Autodesk Inventor part; units mm, degrees
(part 3 of 4)
  arc A595 (24.0109, 33.4184) -> (24.0599, 33.8093) centre (17.6805, 34.4109) ccw
  arc A596 (24.0599, 33.8093) -> (24.09, 34.2945) centre (16.5061, 34.5221) ccw
  arc A597 (24.09, 34.2945) -> (23.7273, 34.4617) centre (15.3265, 15.7621) ccw
  arc A598 (23.7273, 34.4617) -> (23.3779, 34.1237) centre (28.8257, 28.8427) ccw
  arc A599 (23.3779, 34.1237) -> (23.1125, 33.8326) centre (27.9785, 29.6635) ccw
  arc A600 (23.1125, 33.8326) -> (22.9159, 33.5888) centre (27.1156, 30.4021) ccw
  arc A601 (22.9159, 33.5888) -> (22.5655, 33.7339) centre (15.3265, 15.7621) ccw
  arc A602 (22.5655, 33.7339) -> (22.5988, 34.0453) centre (17.3425, 34.4503) ccw
  arc A603 (22.5988, 34.0453) -> (22.617, 34.4389) centre (16.2101, 34.5381) ccw
  arc A604 (22.617, 34.4389) -> (22.609, 34.9249) centre (15.0306, 34.5568) ccw
  arc A605 (22.609, 34.9249) -> (22.2342, 35.0632) centre (15.3265, 15.7621) ccw
  arc A606 (22.2342, 35.0632) -> (21.9125, 34.6988) centre (27.7578, 29.8615) ccw
  arc A607 (21.9125, 34.6988) -> (21.6707, 34.3877) centre (26.8488, 30.6133) ccw
  arc A608 (21.6707, 34.3877) -> (21.4938, 34.1293) centre (25.9306, 31.2819) ccw
  arc A609 (21.4938, 34.1293) -> (21.1331, 34.2465) centre (15.3265, 15.7621) ccw
  arc A610 (21.1331, 34.2465) -> (21.1419, 34.5595) centre (15.87, 34.5508) ccw
  arc A611 (21.1419, 34.5595) -> (21.1292, 34.9533) centre (14.7342, 34.5495) ccw
  arc A612 (21.1292, 34.9533) -> (21.083, 35.4372) centre (13.5569, 34.4756) ccw
  arc A613 (21.083, 35.4372) -> (20.6986, 35.5457) centre (15.3265, 15.7621) ccw
  arc A614 (20.6986, 35.5457) -> (20.4064, 35.1572) centre (26.6132, 30.7934) ccw
  arc A615 (20.4064, 35.1572) -> (20.1898, 34.8281) centre (25.648, 31.4715) ccw
  arc A616 (20.1898, 34.8281) -> (20.0337, 34.5566) centre (24.6803, 32.0661) ccw
  arc A617 (20.0337, 34.5566) -> (19.6649, 34.6451) centre (15.3265, 15.7621) ccw
  arc A618 (19.6649, 34.6451) -> (19.6491, 34.9579) centre (14.3942, 34.5355) ccw
  arc A619 (19.6491, 34.9579) -> (19.6056, 35.3494) centre (13.262, 34.4452) ccw
  arc A620 (19.6056, 35.3494) -> (19.5216, 35.8282) centre (12.0941, 34.2791) ccw
  arc A621 (19.5216, 35.8282) -> (19.1298, 35.9062) centre (15.3265, 15.7621) ccw
  arc A622 (19.1298, 35.9062) -> (18.869, 35.4959) centre (25.3991, 31.6326) ccw
  arc A623 (18.869, 35.4959) -> (18.6789, 35.1509) centre (24.3837, 32.2329) ccw
  arc A624 (18.6789, 35.1509) -> (18.5446, 34.8679) centre (23.3723, 32.7497) ccw
  arc A625 (18.5446, 34.8679) -> (18.17, 34.9273) centre (15.3265, 15.7621) ccw
  arc A626 (18.17, 34.9273) -> (18.1297, 35.2378) centre (12.9241, 34.4045) ccw
  arc A627 (18.1297, 35.2378) -> (18.0556, 35.6248) centre (11.8025, 34.2256) ccw
  arc A628 (18.0556, 35.6248) -> (17.9343, 36.0955) centre (10.6512, 33.9684) ccw
  arc A629 (17.9343, 36.0955) -> (17.5376, 36.1425) centre (15.3265, 15.7621) ccw
  arc A630 (17.5376, 36.1425) -> (17.3098, 35.713) centre (24.1229, 32.3739) ccw
  arc A631 (17.3098, 35.713) -> (17.1473, 35.3541) centre (23.0635, 32.8927) ccw
  arc A632 (17.1473, 35.3541) -> (17.0357, 35.0615) centre (22.0146, 33.3286) ccw
  arc A633 (17.0357, 35.0615) -> (16.6576, 35.0913) centre (15.3265, 15.7621) ccw
  arc A634 (16.6576, 35.0913) -> (16.593, 35.3977) centre (11.4688, 34.1586) ccw
  arc A635 (16.593, 35.3977) -> (16.4887, 35.7777) centre (10.3647, 33.8922) ccw
  arc A636 (16.4887, 35.7777) -> (16.3309, 36.2374) centre (9.2372, 33.5455) ccw
  arc A637 (16.3309, 36.2374) -> (15.9318, 36.2531) centre (15.3265, 15.7621) ccw
  arc A638 (15.9318, 36.2531) -> (15.7383, 35.8071) centre (22.7924, 33.0129) ccw
  arc A639 (15.7383, 35.8071) -> (15.6046, 35.4366) centre (21.6956, 33.447) ccw
  circle A640 centre (15.3265, 15.7621) radius 18.25
  point P0 (0, 0)
  dimension "d2" = 36.5
  constraints: 1 centre point, 1 coincident
  measures "d2" diameter of A640
extrude "押し出し2" cut sketch "スケッチ2" against normal blind 0.75 contours A640
sketch "スケッチ3" plane through (0, 0, 0) normal (0, 0, -1) x (-1, 0, 0)
  arc A0 (-15.5162, 35.1361) -> (-15.6046, 35.4366) centre (-20.6157, 33.7992) ccw
  arc A1 (-15.6046, 35.4366) -> (-15.7383, 35.8071) centre (-21.6956, 33.447) ccw
  arc A2 (-15.7383, 35.8071) -> (-15.9318, 36.2531) centre (-22.7924, 33.0129) ccw
  arc A3 (-15.9318, 36.2531) -> (-16.3309, 36.2374) centre (-15.3265, 15.7621) ccw
  arc A4 (-16.3309, 36.2374) -> (-16.4887, 35.7777) centre (-9.2372, 33.5455) ccw
  arc A5 (-16.4887, 35.7777) -> (-16.593, 35.3977) centre (-10.3647, 33.8922) ccw
  arc A6 (-16.593, 35.3977) -> (-16.6576, 35.0913) centre (-11.4688, 34.1586) ccw
  arc A7 (-16.6576, 35.0913) -> (-17.0357, 35.0615) centre (-15.3265, 15.7621) ccw
  arc A8 (-17.0357, 35.0615) -> (-17.1473, 35.3541) centre (-22.0146, 33.3286) ccw
  arc A9 (-17.1473, 35.3541) -> (-17.3098, 35.713) centre (-23.0635, 32.8927) ccw
  arc A10 (-17.3098, 35.713) -> (-17.5376, 36.1425) centre (-24.1229, 32.3739) ccw
  arc A11 (-17.5376, 36.1425) -> (-17.9343, 36.0955) centre (-15.3265, 15.7621) ccw
  arc A12 (-17.9343, 36.0955) -> (-18.0556, 35.6248) centre (-10.6512, 33.9684) ccw
  arc A13 (-18.0556, 35.6248) -> (-18.1297, 35.2378) centre (-11.8025, 34.2256) ccw
  arc A14 (-18.1297, 35.2378) -> (-18.17, 34.9273) centre (-12.9241, 34.4045) ccw
  arc A15 (-18.17, 34.9273) -> (-18.5446, 34.8679) centre (-15.3265, 15.7621) ccw
  arc A16 (-18.5446, 34.8679) -> (-18.6789, 35.1509) centre (-23.3723, 32.7497) ccw
  arc A17 (-18.6789, 35.1509) -> (-18.869, 35.4959) centre (-24.3837, 32.2329) ccw
  arc A18 (-18.869, 35.4959) -> (-19.1298, 35.9062) centre (-25.3991, 31.6326) ccw
  arc A19 (-19.1298, 35.9062) -> (-19.5216, 35.8282) centre (-15.3265, 15.7621) ccw
  arc A20 (-19.5216, 35.8282) -> (-19.6056, 35.3494) centre (-12.0941, 34.2791) ccw
  arc A21 (-19.6056, 35.3494) -> (-19.6491, 34.9579) centre (-13.262, 34.4452) ccw
  arc A22 (-19.6491, 34.9579) -> (-19.6649, 34.6451) centre (-14.3942, 34.5355) ccw
  arc A23 (-19.6649, 34.6451) -> (-20.0337, 34.5566) centre (-15.3265, 15.7621) ccw
  arc A24 (-20.0337, 34.5566) -> (-20.1898, 34.8281) centre (-24.6803, 32.0661) ccw
  arc A25 (-20.1898, 34.8281) -> (-20.4064, 35.1572) centre (-25.648, 31.4715) ccw
  arc A26 (-20.4064, 35.1572) -> (-20.6986, 35.5457) centre (-26.6132, 30.7934) ccw
  arc A27 (-20.6986, 35.5457) -> (-21.083, 35.4372) centre (-15.3265, 15.7621) ccw
  arc A28 (-21.083, 35.4372) -> (-21.1292, 34.9533) centre (-13.5569, 34.4756) ccw
  arc A29 (-21.1292, 34.9533) -> (-21.1419, 34.5595) centre (-14.7342, 34.5495) ccw
  arc A30 (-21.1419, 34.5595) -> (-21.1331, 34.2465) centre (-15.87, 34.5508) ccw
  arc A31 (-21.1331, 34.2465) -> (-21.4938, 34.1293) centre (-15.3265, 15.7621) ccw
  arc A32 (-21.4938, 34.1293) -> (-21.6707, 34.3877) centre (-25.9306, 31.2819) ccw
  arc A33 (-21.6707, 34.3877) -> (-21.9125, 34.6988) centre (-26.8488, 30.6133) ccw
  arc A34 (-21.9125, 34.6988) -> (-22.2342, 35.0632) centre (-27.7578, 29.8615) ccw
  arc A35 (-22.2342, 35.0632) -> (-22.609, 34.9249) centre (-15.3265, 15.7621) ccw
  arc A36 (-22.609, 34.9249) -> (-22.617, 34.4389) centre (-15.0306, 34.5568) ccw
  arc A37 (-22.617, 34.4389) -> (-22.5988, 34.0453) centre (-16.2101, 34.5381) ccw
  arc A38 (-22.5988, 34.0453) -> (-22.5655, 33.7339) centre (-17.3425, 34.4503) ccw
  arc A39 (-22.5655, 33.7339) -> (-22.9159, 33.5888) centre (-15.3265, 15.7621) ccw
  arc A40 (-22.9159, 33.5888) -> (-23.1125, 33.8326) centre (-27.1156, 30.4021) ccw
  arc A41 (-23.1125, 33.8326) -> (-23.3779, 34.1237) centre (-27.9785, 29.6635) ccw
  arc A42 (-23.3779, 34.1237) -> (-23.7273, 34.4617) centre (-28.8257, 28.8427) ccw
  arc A43 (-23.7273, 34.4617) -> (-24.09, 34.2945) centre (-15.3265, 15.7621) ccw
  arc A44 (-24.09, 34.2945) -> (-24.0599, 33.8093) centre (-16.5061, 34.5221) ccw
  arc A45 (-24.0599, 33.8093) -> (-24.0109, 33.4184) centre (-17.6805, 34.4109) ccw
  arc A46 (-24.0109, 33.4184) -> (-23.9532, 33.1106) centre (-18.8025, 34.2345) ccw
  arc A47 (-23.9532, 33.1106) -> (-24.2911, 32.9384) centre (-15.3265, 15.7621) ccw
  arc A48 (-24.2911, 32.9384) -> (-24.5063, 33.166) centre (-28.2279, 29.432) ccw
  arc A49 (-24.5063, 33.166) -> (-24.7937, 33.4354) centre (-29.0302, 28.628) ccw
  arc A50 (-24.7937, 33.4354) -> (-25.1685, 33.745) centre (-29.8104, 27.7432) ccw
  arc A51 (-25.1685, 33.745) -> (-25.5171, 33.5498) centre (-15.3265, 15.7621) ccw
  arc A52 (-25.5171, 33.5498) -> (-25.449, 33.0685) centre (-17.9744, 34.3717) ccw
  arc A53 (-25.449, 33.0685) -> (-25.3694, 32.6826) centre (-19.1364, 34.1687) ccw
  arc A54 (-25.3694, 32.6826) -> (-25.2878, 32.3803) centre (-20.2411, 33.9048) ccw
  arc A55 (-25.2878, 32.3803) -> (-25.6112, 32.1821) centre (-15.3265, 15.7621) ccw
  arc A56 (-25.6112, 32.1821) -> (-25.8435, 32.3921) centre (-29.2607, 28.3776) ccw
  arc A57 (-25.8435, 32.3921) -> (-26.1512, 32.6381) centre (-29.9974, 27.5131) ccw
  arc A58 (-26.1512, 32.6381) -> (-26.5491, 32.9173) centre (-30.7058, 26.5699) ccw
  arc A59 (-26.5491, 32.9173) -> (-26.8813, 32.6954) centre (-15.3265, 15.7621) ccw
  arc A60 (-26.8813, 32.6954) -> (-26.7756, 32.2209) centre (-19.4263, 34.1066) ccw
  arc A61 (-26.7756, 32.2209) -> (-26.666, 31.8425) centre (-20.5688, 33.8131) ccw
  arc A62 (-26.666, 31.8425) -> (-26.5609, 31.5475) centre (-21.6494, 33.4633) ccw
  arc A63 (-26.5609, 31.5475) -> (-26.8677, 31.3246) centre (-15.3265, 15.7621) ccw
  arc A64 (-26.8677, 31.3246) -> (-27.1158, 31.5157) centre (-30.2075, 27.2455) ccw
  arc A65 (-27.1158, 31.5157) -> (-27.4419, 31.7368) centre (-30.8741, 26.3258) ccw
  arc A66 (-27.4419, 31.7368) -> (-27.8605, 31.984) centre (-31.5063, 25.33) ccw
  arc A67 (-27.8605, 31.984) -> (-28.1742, 31.7366) centre (-15.3265, 15.7621) ccw
  arc A68 (-28.1742, 31.7366) -> (-28.0317, 31.2719) centre (-20.853, 33.7284) ccw
  arc A69 (-28.0317, 31.2719) -> (-27.8927, 30.9032) centre (-21.9689, 33.3461) ccw
  arc A70 (-27.8927, 30.9032) -> (-27.7648, 30.6174) centre (-23.0188, 32.9126) ccw
  arc A71 (-27.7648, 30.6174) -> (-28.0532, 30.3711) centre (-15.3265, 15.7621) ccw
  arc A72 (-28.0532, 30.3711) -> (-28.3155, 30.5421) centre (-31.0626, 26.0425) ccw
  arc A73 (-28.3155, 30.5421) -> (-28.6579, 30.737) centre (-31.655, 25.0734) ccw
  arc A74 (-28.6579, 30.737) -> (-29.0946, 30.9505) centre (-32.2071, 24.031) ccw
  arc A75 (-29.0946, 30.9505) -> (-29.388, 30.6794) centre (-15.3265, 15.7621) ccw
  arc A76 (-29.388, 30.6794) -> (-29.2094, 30.2273) centre (-22.2456, 33.2394) ccw
  arc A77 (-29.2094, 30.2273) -> (-29.0419, 29.8706) centre (-23.3281, 32.7708) ccw
  arc A78 (-29.0419, 29.8706) -> (-28.892, 29.5957) centre (-24.3407, 32.2563) ccw
  arc A79 (-28.892, 29.5957) -> (-29.1602, 29.3275) centre (-15.3265, 15.7621) ccw
  arc A80 (-29.1602, 29.3275) -> (-29.4351, 29.4775) centre (-31.8207, 24.7762) ccw
  arc A81 (-29.4351, 29.4775) -> (-29.7917, 29.6449) centre (-32.3352, 23.7636) ccw
  arc A82 (-29.7917, 29.6449) -> (-30.2439, 29.8235) centre (-32.8039, 22.6811) ccw
  arc A83 (-30.2439, 29.8235) -> (-30.515, 29.5302) centre (-15.3265, 15.7621) ccw
  arc A84 (-30.515, 29.5302) -> (-30.3015, 29.0934) centre (-23.5955, 32.6427) ccw
  arc A85 (-30.3015, 29.0934) -> (-30.1066, 28.751) centre (-24.6379, 32.0905) ccw
  arc A86 (-30.1066, 28.751) -> (-29.9356, 28.4887) centre (-25.607, 31.4982) ccw
  arc A87 (-29.9356, 28.4887) -> (-30.1819, 28.2003) centre (-15.3265, 15.7621) ccw
  arc A88 (-30.1819, 28.2003) -> (-30.4677, 28.3282) centre (-32.4771, 23.4543) ccw
  arc A89 (-30.4677, 28.3282) -> (-30.8364, 28.4672) centre (-32.9106, 22.4045) ccw
  arc A90 (-30.8364, 28.4672) -> (-31.3011, 28.6097) centre (-33.2929, 21.2885) ccw
  arc A91 (-31.3011, 28.6097) -> (-31.5484, 28.296) centre (-15.3265, 15.7621) ccw
  arc A92 (-31.5484, 28.296) -> (-31.3013, 27.8774) centre (-24.8944, 31.9418) ccw
  arc A93 (-31.3013, 27.8774) -> (-31.0801, 27.5514) centre (-25.8903, 31.3096) ccw
  arc A94 (-31.0801, 27.5514) -> (-30.889, 27.3033) centre (-26.81, 30.6431) ccw
  arc A95 (-30.889, 27.3033) -> (-31.112, 26.9964) centre (-15.3265, 15.7621) ccw
  arc A96 (-31.112, 26.9964) -> (-31.407, 27.1015) centre (-33.0278, 22.085) ccw
  arc A97 (-31.407, 27.1015) -> (-31.7854, 27.2111) centre (-33.3775, 21.0044) ccw
  arc A98 (-31.7854, 27.2111) -> (-32.2599, 27.3168) centre (-33.6711, 19.8618) ccw
  arc A99 (-32.2599, 27.3168) -> (-32.4818, 26.9846) centre (-15.3265, 15.7621) ccw
  arc A100 (-32.4818, 26.9846) -> (-32.2026, 26.5867) centre (-26.1344, 31.1413) ccw
  arc A101 (-32.2026, 26.5867) -> (-31.9566, 26.279) centre (-27.0776, 30.4329) ccw
  arc A102 (-31.9566, 26.279) -> (-31.7466, 26.0467) centre (-27.9421, 29.6962) ccw
  arc A103 (-31.7466, 26.0467) -> (-31.9447, 25.7233) centre (-15.3265, 15.7621) ccw
  arc A104 (-31.9447, 25.7233) -> (-32.2471, 25.8049) centre (-33.4693, 20.6766) ccw
  arc A105 (-32.2471, 25.8049) -> (-32.633, 25.8845) centre (-33.7332, 19.5719) ccw
  arc A106 (-32.633, 25.8845) -> (-33.1143, 25.9526) centre (-33.9362, 18.4099) ccw
  arc A107 (-33.1143, 25.9526) -> (-33.3095, 25.6041) centre (-15.3265, 15.7621) ccw
  arc A108 (-33.3095, 25.6041) -> (-32.9999, 25.2293) centre (-27.3077, 30.2459) ccw
  arc A109 (-32.9999, 25.2293) -> (-32.7304, 24.9418) centre (-28.1924, 29.4657) ccw
  arc A110 (-32.7304, 24.9418) -> (-32.5029, 24.7267) centre (-28.9965, 28.6635) ccw
  arc A111 (-32.5029, 24.7267) -> (-32.6751, 24.3888) centre (-15.3265, 15.7621) ccw
  arc A112 (-32.6751, 24.3888) -> (-32.9829, 24.4464) centre (-33.799, 19.238) ccw
  arc A113 (-32.9829, 24.4464) -> (-33.3738, 24.4954) centre (-33.9754, 18.116) ccw
  arc A114 (-33.3738, 24.4954) -> (-33.859, 24.5256) centre (-34.0866, 16.9417) ccw
  arc A115 (-33.859, 24.5256) -> (-34.0262, 24.1628) centre (-15.3265, 15.7621) ccw
  arc A116 (-34.0262, 24.1628) -> (-33.6882, 23.8134) centre (-28.4072, 29.2612) ccw
  arc A117 (-33.6882, 23.8134) -> (-33.397, 23.548) centre (-29.228, 28.414) ccw
  arc A118 (-33.397, 23.548) -> (-33.1533, 23.3514) centre (-29.9666, 27.5512) ccw
  arc A119 (-33.1533, 23.3514) -> (-33.2984, 23.001) centre (-15.3265, 15.7621) ccw
  arc A120 (-33.2984, 23.001) -> (-33.6098, 23.0343) centre (-34.0147, 17.778) ccw
  arc A121 (-33.6098, 23.0343) -> (-34.0034, 23.0525) centre (-34.1026, 16.6456) ccw
  arc A122 (-34.0034, 23.0525) -> (-34.4894, 23.0445) centre (-34.1213, 15.4661) ccw
  arc A123 (-34.4894, 23.0445) -> (-34.6277, 22.6697) centre (-15.3265, 15.7621) ccw
  arc A124 (-34.6277, 22.6697) -> (-34.2633, 22.348) centre (-29.426, 28.1933) ccw
  arc A125 (-34.2633, 22.348) -> (-33.9522, 22.1062) centre (-30.1778, 27.2843) ccw
  arc A126 (-33.9522, 22.1062) -> (-33.6938, 21.9293) centre (-30.8464, 26.3662) ccw
  arc A127 (-33.6938, 21.9293) -> (-33.811, 21.5686) centre (-15.3265, 15.7621) ccw
  arc A128 (-33.811, 21.5686) -> (-34.124, 21.5774) centre (-34.1153, 16.3055) ccw
  arc A129 (-34.124, 21.5774) -> (-34.5178, 21.5647) centre (-34.114, 15.1697) ccw
  arc A130 (-34.5178, 21.5647) -> (-35.0017, 21.5186) centre (-34.0401, 13.9924) ccw
  arc A131 (-35.0017, 21.5186) -> (-35.1102, 21.1341) centre (-15.3265, 15.7621) ccw
  arc A132 (-35.1102, 21.1341) -> (-34.7216, 20.8419) centre (-30.3579, 27.0488) ccw
  arc A133 (-34.7216, 20.8419) -> (-34.3925, 20.6253) centre (-31.036, 26.0836) ccw
  arc A134 (-34.3925, 20.6253) -> (-34.121, 20.4692) centre (-31.6305, 25.1158) ccw
  arc A135 (-34.121, 20.4692) -> (-34.2096, 20.1005) centre (-15.3265, 15.7621) ccw
  arc A136 (-34.2096, 20.1005) -> (-34.5223, 20.0847) centre (-34.1, 14.8297) ccw
  arc A137 (-34.5223, 20.0847) -> (-34.9139, 20.0411) centre (-34.0096, 13.6975) ccw
  arc A138 (-34.9139, 20.0411) -> (-35.3927, 19.9571) centre (-33.8436, 12.5296) ccw
  arc A139 (-35.3927, 19.9571) -> (-35.4707, 19.5653) centre (-15.3265, 15.7621) ccw
  arc A140 (-35.4707, 19.5653) -> (-35.0604, 19.3045) centre (-31.1971, 25.8346) ccw
  arc A141 (-35.0604, 19.3045) -> (-34.7153, 19.1144) centre (-31.7974, 24.8192) ccw
  arc A142 (-34.7153, 19.1144) -> (-34.4324, 18.9801) centre (-32.3142, 23.8078) ccw
  arc A143 (-34.4324, 18.9801) -> (-34.4918, 18.6055) centre (-15.3265, 15.7621) ccw
  arc A144 (-34.4918, 18.6055) -> (-34.8023, 18.5653) centre (-33.969, 13.3596) ccw
  arc A145 (-34.8023, 18.5653) -> (-35.1893, 18.4911) centre (-33.7901, 12.238) ccw
  arc A146 (-35.1893, 18.4911) -> (-35.66, 18.3698) centre (-33.5329, 11.0868) ccw
  arc A147 (-35.66, 18.3698) -> (-35.707, 17.9731) centre (-15.3265, 15.7621) ccw
  arc A148 (-35.707, 17.9731) -> (-35.2775, 17.7453) centre (-31.9384, 24.5584) ccw
  arc A149 (-35.2775, 17.7453) -> (-34.9186, 17.5829) centre (-32.4572, 23.499) ccw
  arc A150 (-34.9186, 17.5829) -> (-34.626, 17.4712) centre (-32.8931, 22.4501) ccw
  arc A151 (-34.626, 17.4712) -> (-34.6558, 17.0931) centre (-15.3265, 15.7621) ccw
  arc A152 (-34.6558, 17.0931) -> (-34.9622, 17.0286) centre (-33.723, 11.9043) ccw
  arc A153 (-34.9622, 17.0286) -> (-35.3421, 16.9243) centre (-33.4566, 10.8002) ccw
  arc A154 (-35.3421, 16.9243) -> (-35.8019, 16.7664) centre (-33.11, 9.6727) ccw
  arc A155 (-35.8019, 16.7664) -> (-35.8176, 16.3673) centre (-15.3265, 15.7621) ccw
  arc A156 (-35.8176, 16.3673) -> (-35.3716, 16.1739) centre (-32.5774, 23.2279) ccw
  arc A157 (-35.3716, 16.1739) -> (-35.0011, 16.0401) centre (-33.0115, 22.1311) ccw
  arc A158 (-35.0011, 16.0401) -> (-34.7006, 15.9517) centre (-33.3636, 21.0513) ccw
  arc A159 (-34.7006, 15.9517) -> (-34.7006, 15.5724) centre (-15.3265, 15.7621) ccw
  arc A160 (-34.7006, 15.5724) -> (-35.0011, 15.4841) centre (-33.3636, 10.4729) ccw
  arc A161 (-35.0011, 15.4841) -> (-35.3716, 15.3503) centre (-33.0115, 9.3931) ccw
  arc A162 (-35.3716, 15.3503) -> (-35.8176, 15.1569) centre (-32.5774, 8.2962) ccw
  arc A163 (-35.8176, 15.1569) -> (-35.8019, 14.7577) centre (-15.3265, 15.7621) ccw
  arc A164 (-35.8019, 14.7577) -> (-35.3421, 14.5999) centre (-33.11, 21.8514) ccw
  arc A165 (-35.3421, 14.5999) -> (-34.9622, 14.4956) centre (-33.4566, 20.7239) ccw
  arc A166 (-34.9622, 14.4956) -> (-34.6558, 14.431) centre (-33.723, 19.6198) ccw
  arc A167 (-34.6558, 14.431) -> (-34.626, 14.053) centre (-15.3265, 15.7621) ccw
  arc A168 (-34.626, 14.053) -> (-34.9186, 13.9413) centre (-32.8931, 9.074) ccw
  arc A169 (-34.9186, 13.9413) -> (-35.2775, 13.7788) centre (-32.4572, 8.0251) ccw
  arc A170 (-35.2775, 13.7788) -> (-35.707, 13.551) centre (-31.9384, 6.9657) ccw
  arc A171 (-35.707, 13.551) -> (-35.66, 13.1543) centre (-15.3265, 15.7621) ccw
  arc A172 (-35.66, 13.1543) -> (-35.1893, 13.033) centre (-33.5329, 20.4374) ccw
  arc A173 (-35.1893, 13.033) -> (-34.8023, 12.9589) centre (-33.7901, 19.2861) ccw
  arc A174 (-34.8023, 12.9589) -> (-34.4918, 12.9186) centre (-33.969, 18.1645) ccw
  arc A175 (-34.4918, 12.9186) -> (-34.4324, 12.544) centre (-15.3265, 15.7621) ccw
  arc A176 (-34.4324, 12.544) -> (-34.7153, 12.4097) centre (-32.3142, 7.7164) ccw
  arc A177 (-34.7153, 12.4097) -> (-35.0604, 12.2196) centre (-31.7974, 6.7049) ccw
  arc A178 (-35.0604, 12.2196) -> (-35.4707, 11.9588) centre (-31.1971, 5.6895) ccw
  arc A179 (-35.4707, 11.9588) -> (-35.3927, 11.567) centre (-15.3265, 15.7621) ccw
  arc A180 (-35.3927, 11.567) -> (-34.9139, 11.4831) centre (-33.8436, 18.9945) ccw
  arc A181 (-34.9139, 11.4831) -> (-34.5223, 11.4395) centre (-34.0096, 17.8266) ccw
  arc A182 (-34.5223, 11.4395) -> (-34.2096, 11.4237) centre (-34.1, 16.6945) ccw
  arc A183 (-34.2096, 11.4237) -> (-34.121, 11.0549) centre (-15.3265, 15.7621) ccw
  arc A184 (-34.121, 11.0549) -> (-34.3925, 10.8988) centre (-31.6305, 6.4083) ccw
  arc A185 (-34.3925, 10.8988) -> (-34.7216, 10.6822) centre (-31.036, 5.4406) ccw
  arc A186 (-34.7216, 10.6822) -> (-35.1102, 10.39) centre (-30.3579, 4.4754) ccw
  arc A187 (-35.1102, 10.39) -> (-35.0017, 10.0056) centre (-15.3265, 15.7621) ccw
  arc A188 (-35.0017, 10.0056) -> (-34.5178, 9.9594) centre (-34.0401, 17.5317) ccw
  arc A189 (-34.5178, 9.9594) -> (-34.124, 9.9467) centre (-34.114, 16.3544) ccw
  arc A190 (-34.124, 9.9467) -> (-33.811, 9.9555) centre (-34.1153, 15.2186) ccw
  arc A191 (-33.811, 9.9555) -> (-33.6938, 9.5948) centre (-15.3265, 15.7621) ccw
  arc A192 (-33.6938, 9.5948) -> (-33.9522, 9.4179) centre (-30.8464, 5.158) ccw
  arc A193 (-33.9522, 9.4179) -> (-34.2633, 9.1762) centre (-30.1778, 4.2398) ccw
  arc A194 (-34.2633, 9.1762) -> (-34.6277, 8.8544) centre (-29.426, 3.3308) ccw
  arc A195 (-34.6277, 8.8544) -> (-34.4894, 8.4796) centre (-15.3265, 15.7621) ccw
  arc A196 (-34.4894, 8.4796) -> (-34.0034, 8.4716) centre (-34.1213, 16.058) ccw
  arc A197 (-34.0034, 8.4716) -> (-33.6098, 8.4898) centre (-34.1026, 14.8785) ccw
  arc A198 (-33.6098, 8.4898) -> (-33.2984, 8.5231) centre (-34.0147, 13.7462) ccw
  arc A199 (-33.2984, 8.5231) -> (-33.1533, 8.1727) centre (-15.3265, 15.7621) ccw
  arc A200 (-33.1533, 8.1727) -> (-33.397, 7.9761) centre (-29.9666, 3.973) ccw
  arc A201 (-33.397, 7.9761) -> (-33.6882, 7.7107) centre (-29.228, 3.1101) ccw
  arc A202 (-33.6882, 7.7107) -> (-34.0262, 7.3613) centre (-28.4072, 2.2629) ccw
  arc A203 (-34.0262, 7.3613) -> (-33.859, 6.9986) centre (-15.3265, 15.7621) ccw
  arc A204 (-33.859, 6.9986) -> (-33.3738, 7.0287) centre (-34.0866, 14.5825) ccw
  arc A205 (-33.3738, 7.0287) -> (-32.9829, 7.0777) centre (-33.9754, 13.4081) ccw
  arc A206 (-32.9829, 7.0777) -> (-32.6751, 7.1354) centre (-33.799, 12.2861) ccw
  arc A207 (-32.6751, 7.1354) -> (-32.5029, 6.7975) centre (-15.3265, 15.7621) ccw
  arc A208 (-32.5029, 6.7975) -> (-32.7304, 6.5823) centre (-28.9965, 2.8607) ccw
  arc A209 (-32.7304, 6.5823) -> (-32.9999, 6.2949) centre (-28.1924, 2.0585) ccw
  arc A210 (-32.9999, 6.2949) -> (-33.3095, 5.9201) centre (-27.3077, 1.2782) ccw
  arc A211 (-33.3095, 5.9201) -> (-33.1143, 5.5715) centre (-15.3265, 15.7621) ccw
  arc A212 (-33.1143, 5.5715) -> (-32.633, 5.6397) centre (-33.9362, 13.1142) ccw
  arc A213 (-32.633, 5.6397) -> (-32.2471, 5.7192) centre (-33.7332, 11.9522) ccw
  arc A214 (-32.2471, 5.7192) -> (-31.9447, 5.8008) centre (-33.4693, 10.8475) ccw
  arc A215 (-31.9447, 5.8008) -> (-31.7466, 5.4775) centre (-15.3265, 15.7621) ccw
  arc A216 (-31.7466, 5.4775) -> (-31.9566, 5.2451) centre (-27.9421, 1.8279) ccw
  arc A217 (-31.9566, 5.2451) -> (-32.2026, 4.9374) centre (-27.0776, 1.0913) ccw
  arc A218 (-32.2026, 4.9374) -> (-32.4818, 4.5395) centre (-26.1344, 0.3829) ccw
  arc A219 (-32.4818, 4.5395) -> (-32.2599, 4.2073) centre (-15.3265, 15.7621) ccw
  arc A220 (-32.2599, 4.2073) -> (-31.7854, 4.313) centre (-33.6711, 11.6623) ccw
  arc A221 (-31.7854, 4.313) -> (-31.407, 4.4226) centre (-33.3775, 10.5198) ccw
  arc A222 (-31.407, 4.4226) -> (-31.112, 4.5277) centre (-33.0278, 9.4392) ccw
  arc A223 (-31.112, 4.5277) -> (-30.889, 4.2209) centre (-15.3265, 15.7621) ccw
  arc A224 (-30.889, 4.2209) -> (-31.0801, 3.9728) centre (-26.81, 0.8811) ccw
  arc A225 (-31.0801, 3.9728) -> (-31.3013, 3.6467) centre (-25.8903, 0.2145) ccw
  arc A226 (-31.3013, 3.6467) -> (-31.5484, 3.2281) centre (-24.8944, -0.4177) ccw
  arc A227 (-31.5484, 3.2281) -> (-31.3011, 2.9144) centre (-15.3265, 15.7621) ccw
  arc A228 (-31.3011, 2.9144) -> (-30.8364, 3.057) centre (-33.2929, 10.2356) ccw
  arc A229 (-30.8364, 3.057) -> (-30.4677, 3.1959) centre (-32.9106, 9.1197) ccw
  arc A230 (-30.4677, 3.1959) -> (-30.1819, 3.3238) centre (-32.4771, 8.0698) ccw
  arc A231 (-30.1819, 3.3238) -> (-29.9356, 3.0354) centre (-15.3265, 15.7621) ccw
  arc A232 (-29.9356, 3.0354) -> (-30.1066, 2.7731) centre (-25.607, 0.026) ccw
  arc A233 (-30.1066, 2.7731) -> (-30.3015, 2.4307) centre (-24.6379, -0.5664) ccw
  arc A234 (-30.3015, 2.4307) -> (-30.515, 1.994) centre (-23.5955, -1.1185) ccw
  arc A235 (-30.515, 1.994) -> (-30.2439, 1.7006) centre (-15.3265, 15.7621) ccw
  arc A236 (-30.2439, 1.7006) -> (-29.7917, 1.8792) centre (-32.8039, 8.843) ccw
  arc A237 (-29.7917, 1.8792) -> (-29.4351, 2.0467) centre (-32.3352, 7.7605) ccw
  arc A238 (-29.4351, 2.0467) -> (-29.1602, 2.1966) centre (-31.8207, 6.7479) ccw
  arc A239 (-29.1602, 2.1966) -> (-28.892, 1.9284) centre (-15.3265, 15.7621) ccw
  arc A240 (-28.892, 1.9284) -> (-29.0419, 1.6535) centre (-24.3407, -0.7321) ccw
  arc A241 (-29.0419, 1.6535) -> (-29.2094, 1.2969) centre (-23.3281, -1.2466) ccw
  arc A242 (-29.2094, 1.2969) -> (-29.388, 0.8447) centre (-22.2456, -1.7153) ccw
  arc A243 (-29.388, 0.8447) -> (-29.0946, 0.5736) centre (-15.3265, 15.7621) ccw
  arc A244 (-29.0946, 0.5736) -> (-28.6579, 0.7871) centre (-32.2071, 7.4931) ccw
  arc A245 (-28.6579, 0.7871) -> (-28.3155, 0.982) centre (-31.655, 6.4507) ccw
  arc A246 (-28.3155, 0.982) -> (-28.0532, 1.1531) centre (-31.0626, 5.4816) ccw
  arc A247 (-28.0532, 1.1531) -> (-27.7648, 0.9068) centre (-15.3265, 15.7621) ccw
  arc A248 (-27.7648, 0.9068) -> (-27.8927, 0.6209) centre (-23.0188, -1.3885) ccw
  arc A249 (-27.8927, 0.6209) -> (-28.0317, 0.2522) centre (-21.9689, -1.822) ccw
  arc A250 (-28.0317, 0.2522) -> (-28.1742, -0.2125) centre (-20.853, -2.2042) ccw
  arc A251 (-28.1742, -0.2125) -> (-27.8605, -0.4598) centre (-15.3265, 15.7621) ccw
  arc A252 (-27.8605, -0.4598) -> (-27.4419, -0.2127) centre (-31.5063, 6.1942) ccw
  arc A253 (-27.4419, -0.2127) -> (-27.1158, 0.0085) centre (-30.8741, 5.1983) ccw
  arc A254 (-27.1158, 0.0085) -> (-26.8677, 0.1996) centre (-30.2075, 4.2787) ccw
  arc A255 (-26.8677, 0.1996) -> (-26.5609, -0.0233) centre (-15.3265, 15.7621) ccw
  arc A256 (-26.5609, -0.0233) -> (-26.666, -0.3184) centre (-21.6494, -1.9392) ccw
  arc A257 (-26.666, -0.3184) -> (-26.7756, -0.6968) centre (-20.5688, -2.2889) ccw
  arc A258 (-26.7756, -0.6968) -> (-26.8813, -1.1713) centre (-19.4263, -2.5825) ccw
  arc A259 (-26.8813, -1.1713) -> (-26.5491, -1.3932) centre (-15.3265, 15.7621) ccw
  arc A260 (-26.5491, -1.3932) -> (-26.1512, -1.114) centre (-30.7058, 4.9542) ccw
  arc A261 (-26.1512, -1.114) -> (-25.8435, -0.868) centre (-29.9974, 4.011) ccw
  arc A262 (-25.8435, -0.868) -> (-25.6112, -0.658) centre (-29.2607, 3.1465) ccw
  arc A263 (-25.6112, -0.658) -> (-25.2878, -0.8561) centre (-15.3265, 15.7621) ccw
  arc A264 (-25.2878, -0.8561) -> (-25.3694, -1.1585) centre (-20.2411, -2.3807) ccw
  arc A265 (-25.3694, -1.1585) -> (-25.449, -1.5443) centre (-19.1364, -2.6446) ccw
  arc A266 (-25.449, -1.5443) -> (-25.5171, -2.0257) centre (-17.9744, -2.8476) ccw
  arc A267 (-25.5171, -2.0257) -> (-25.1685, -2.2208) centre (-15.3265, 15.7621) ccw
  arc A268 (-25.1685, -2.2208) -> (-24.7937, -1.9113) centre (-29.8104, 3.7809) ccw
  arc A269 (-24.7937, -1.9113) -> (-24.5063, -1.6418) centre (-29.0302, 2.8962) ccw
  arc A270 (-24.5063, -1.6418) -> (-24.2911, -1.4143) centre (-28.2279, 2.0921) ccw
  arc A271 (-24.2911, -1.4143) -> (-23.9532, -1.5864) centre (-15.3265, 15.7621) ccw
  arc A272 (-23.9532, -1.5864) -> (-24.0109, -1.8943) centre (-18.8025, -2.7104) ccw
  arc A273 (-24.0109, -1.8943) -> (-24.0599, -2.2852) centre (-17.6805, -2.8868) ccw
  arc A274 (-24.0599, -2.2852) -> (-24.09, -2.7704) centre (-16.5061, -2.998) ccw
  arc A275 (-24.09, -2.7704) -> (-23.7273, -2.9376) centre (-15.3265, 15.7621) ccw
  arc A276 (-23.7273, -2.9376) -> (-23.3779, -2.5996) centre (-28.8257, 2.6814) ccw
  arc A277 (-23.3779, -2.5996) -> (-23.1125, -2.3084) centre (-27.9785, 1.8607) ccw
  arc A278 (-23.1125, -2.3084) -> (-22.9159, -2.0647) centre (-27.1156, 1.122) ccw
  arc A279 (-22.9159, -2.0647) -> (-22.5655, -2.2098) centre (-15.3265, 15.7621) ccw
  arc A280 (-22.5655, -2.2098) -> (-22.5988, -2.5212) centre (-17.3425, -2.9261) ccw
  arc A281 (-22.5988, -2.5212) -> (-22.617, -2.9148) centre (-16.2101, -3.014) ccw
  arc A282 (-22.617, -2.9148) -> (-22.609, -3.4008) centre (-15.0306, -3.0327) ccw
  arc A283 (-22.609, -3.4008) -> (-22.2342, -3.5391) centre (-15.3265, 15.7621) ccw
  arc A284 (-22.2342, -3.5391) -> (-21.9125, -3.1747) centre (-27.7578, 1.6626) ccw
  arc A285 (-21.9125, -3.1747) -> (-21.6707, -2.8636) centre (-26.8488, 0.9109) ccw
  arc A286 (-21.6707, -2.8636) -> (-21.4938, -2.6052) centre (-25.9306, 0.2422) ccw
  arc A287 (-21.4938, -2.6052) -> (-21.1331, -2.7224) centre (-15.3265, 15.7621) ccw
  arc A288 (-21.1331, -2.7224) -> (-21.1419, -3.0354) centre (-15.87, -3.0267) ccw
  arc A289 (-21.1419, -3.0354) -> (-21.1292, -3.4292) centre (-14.7342, -3.0254) ccw
  arc A290 (-21.1292, -3.4292) -> (-21.083, -3.9131) centre (-13.5569, -2.9515) ccw
  arc A291 (-21.083, -3.9131) -> (-20.6986, -4.0215) centre (-15.3265, 15.7621) ccw
  arc A292 (-20.6986, -4.0215) -> (-20.4064, -3.633) centre (-26.6132, 0.7308) ccw
  arc A293 (-20.4064, -3.633) -> (-20.1898, -3.3039) centre (-25.648, 0.0526) ccw
  arc A294 (-20.1898, -3.3039) -> (-20.0337, -3.0324) centre (-24.6803, -0.5419) ccw
  arc A295 (-20.0337, -3.0324) -> (-19.6649, -3.121) centre (-15.3265, 15.7621) ccw
  arc A296 (-19.6649, -3.121) -> (-19.6491, -3.4337) centre (-14.3942, -3.0114) ccw
  arc A297 (-19.6491, -3.4337) -> (-19.6056, -3.8253) centre (-13.262, -2.921) ccw
  arc A298 (-19.6056, -3.8253) -> (-19.5216, -4.3041) centre (-12.0941, -2.755) ccw
  arc A299 (-19.5216, -4.3041) -> (-19.1298, -4.382) centre (-15.3265, 15.7621) ccw
  arc A300 (-19.1298, -4.382) -> (-18.869, -3.9718) centre (-25.3991, -0.1085) ccw
  arc A301 (-18.869, -3.9718) -> (-18.6789, -3.6267) centre (-24.3837, -0.7088) ccw
  arc A302 (-18.6789, -3.6267) -> (-18.5446, -3.3438) centre (-23.3723, -1.2256) ccw
  arc A303 (-18.5446, -3.3438) -> (-18.17, -3.4031) centre (-15.3265, 15.7621) ccw
  arc A304 (-18.17, -3.4031) -> (-18.1297, -3.7137) centre (-12.9241, -2.8804) ccw
  arc A305 (-18.1297, -3.7137) -> (-18.0556, -4.1006) centre (-11.8025, -2.7014) ccw
  arc A306 (-18.0556, -4.1006) -> (-17.9343, -4.5714) centre (-10.6512, -2.4443) ccw
  arc A307 (-17.9343, -4.5714) -> (-17.5376, -4.6183) centre (-15.3265, 15.7621) ccw
  arc A308 (-17.5376, -4.6183) -> (-17.3098, -4.1889) centre (-24.1229, -0.8498) ccw
  arc A309 (-17.3098, -4.1889) -> (-17.1473, -3.83) centre (-23.0635, -1.3686) ccw
  arc A310 (-17.1473, -3.83) -> (-17.0357, -3.5374) centre (-22.0146, -1.8045) ccw
  arc A311 (-17.0357, -3.5374) -> (-16.6576, -3.5672) centre (-15.3265, 15.7621) ccw
  arc A312 (-16.6576, -3.5672) -> (-16.593, -3.8736) centre (-11.4688, -2.6344) ccw
  arc A313 (-16.593, -3.8736) -> (-16.4887, -4.2535) centre (-10.3647, -2.368) ccw
  arc A314 (-16.4887, -4.2535) -> (-16.3309, -4.7133) centre (-9.2372, -2.0213) ccw
  arc A315 (-16.3309, -4.7133) -> (-15.9318, -4.729) centre (-15.3265, 15.7621) ccw
  arc A316 (-15.9318, -4.729) -> (-15.7383, -4.283) centre (-22.7924, -1.4888) ccw
  arc A317 (-15.7383, -4.283) -> (-15.6046, -3.9124) centre (-21.6956, -1.9228) ccw
  arc A318 (-15.6046, -3.9124) -> (-15.5162, -3.612) centre (-20.6157, -2.275) ccw
  arc A319 (-15.5162, -3.612) -> (-15.1369, -3.612) centre (-15.3265, 15.7621) ccw
  arc A320 (-15.1369, -3.612) -> (-15.0485, -3.9124) centre (-10.0373, -2.275) ccw
  arc A321 (-15.0485, -3.9124) -> (-14.9147, -4.283) centre (-8.9575, -1.9228) ccw
  arc A322 (-14.9147, -4.283) -> (-14.7213, -4.729) centre (-7.8607, -1.4888) ccw
  arc A323 (-14.7213, -4.729) -> (-14.3222, -4.7133) centre (-15.3265, 15.7621) ccw
  arc A324 (-14.3222, -4.7133) -> (-14.1644, -4.2535) centre (-21.4159, -2.0213) ccw
  arc A325 (-14.1644, -4.2535) -> (-14.0601, -3.8736) centre (-20.2884, -2.368) ccw
  arc A326 (-14.0601, -3.8736) -> (-13.9955, -3.5672) centre (-19.1843, -2.6344) ccw
  arc A327 (-13.9955, -3.5672) -> (-13.6174, -3.5374) centre (-15.3265, 15.7621) ccw
  arc A328 (-13.6174, -3.5374) -> (-13.5057, -3.83) centre (-8.6385, -1.8045) ccw
  arc A329 (-13.5057, -3.83) -> (-13.3433, -4.1889) centre (-7.5896, -1.3686) ccw
  arc A330 (-13.3433, -4.1889) -> (-13.1155, -4.6183) centre (-6.5302, -0.8498) ccw
  arc A331 (-13.1155, -4.6183) -> (-12.7188, -4.5714) centre (-15.3265, 15.7621) ccw
  arc A332 (-12.7188, -4.5714) -> (-12.5975, -4.1006) centre (-20.0019, -2.4443) ccw
  arc A333 (-12.5975, -4.1006) -> (-12.5234, -3.7137) centre (-18.8506, -2.7014) ccw
  arc A334 (-12.5234, -3.7137) -> (-12.4831, -3.4031) centre (-17.729, -2.8804) ccw
  arc A335 (-12.4831, -3.4031) -> (-12.1085, -3.3438) centre (-15.3265, 15.7621) ccw
  arc A336 (-12.1085, -3.3438) -> (-11.9742, -3.6267) centre (-7.2808, -1.2256) ccw
  arc A337 (-11.9742, -3.6267) -> (-11.7841, -3.9718) centre (-6.2694, -0.7088) ccw
  arc A338 (-11.7841, -3.9718) -> (-11.5233, -4.382) centre (-5.254, -0.1085) ccw
  arc A339 (-11.5233, -4.382) -> (-11.1315, -4.3041) centre (-15.3265, 15.7621) ccw
  arc A340 (-11.1315, -4.3041) -> (-11.0475, -3.8253) centre (-18.559, -2.755) ccw
  arc A341 (-11.0475, -3.8253) -> (-11.0039, -3.4337) centre (-17.3911, -2.921) ccw
  arc A342 (-11.0039, -3.4337) -> (-10.9881, -3.121) centre (-16.2589, -3.0114) ccw
  arc A343 (-10.9881, -3.121) -> (-10.6194, -3.0324) centre (-15.3265, 15.7621) ccw
  arc A344 (-10.6194, -3.0324) -> (-10.4633, -3.3039) centre (-5.9728, -0.5419) ccw
  arc A345 (-10.4633, -3.3039) -> (-10.2467, -3.633) centre (-5.005, 0.0526) ccw
  arc A346 (-10.2467, -3.633) -> (-9.9545, -4.0215) centre (-4.0399, 0.7308) ccw
  arc A347 (-9.9545, -4.0215) -> (-9.57, -3.9131) centre (-15.3265, 15.7621) ccw
  arc A348 (-9.57, -3.9131) -> (-9.5239, -3.4292) centre (-17.0962, -2.9515) ccw
  arc A349 (-9.5239, -3.4292) -> (-9.5112, -3.0354) centre (-15.9189, -3.0254) ccw
  arc A350 (-9.5112, -3.0354) -> (-9.52, -2.7224) centre (-14.7831, -3.0267) ccw
  arc A351 (-9.52, -2.7224) -> (-9.1593, -2.6052) centre (-15.3265, 15.7621) ccw
  arc A352 (-9.1593, -2.6052) -> (-8.9824, -2.8636) centre (-4.7224, 0.2422) ccw
  arc A353 (-8.9824, -2.8636) -> (-8.7406, -3.1747) centre (-3.8043, 0.9109) ccw
  arc A354 (-8.7406, -3.1747) -> (-8.4189, -3.5391) centre (-2.8953, 1.6626) ccw
  arc A355 (-8.4189, -3.5391) -> (-8.0441, -3.4008) centre (-15.3265, 15.7621) ccw
  arc A356 (-8.0441, -3.4008) -> (-8.0361, -2.9148) centre (-15.6225, -3.0327) ccw
  arc A357 (-8.0361, -2.9148) -> (-8.0543, -2.5212) centre (-14.443, -3.014) ccw
  arc A358 (-8.0543, -2.5212) -> (-8.0876, -2.2098) centre (-13.3106, -2.9261) ccw
  arc A359 (-8.0876, -2.2098) -> (-7.7372, -2.0647) centre (-15.3265, 15.7621) ccw
  arc A360 (-7.7372, -2.0647) -> (-7.5406, -2.3084) centre (-3.5375, 1.122) ccw
  arc A361 (-7.5406, -2.3084) -> (-7.2752, -2.5996) centre (-2.6746, 1.8607) ccw
  arc A362 (-7.2752, -2.5996) -> (-6.9258, -2.9376) centre (-1.8274, 2.6814) ccw
  arc A363 (-6.9258, -2.9376) -> (-6.563, -2.7704) centre (-15.3265, 15.7621) ccw
  arc A364 (-6.563, -2.7704) -> (-6.5932, -2.2852) centre (-14.147, -2.998) ccw
  arc A365 (-6.5932, -2.2852) -> (-6.6422, -1.8943) centre (-12.9726, -2.8868) ccw
  arc A366 (-6.6422, -1.8943) -> (-6.6999, -1.5864) centre (-11.8506, -2.7104) ccw
  arc A367 (-6.6999, -1.5864) -> (-6.3619, -1.4143) centre (-15.3265, 15.7621) ccw
  arc A368 (-6.3619, -1.4143) -> (-6.1468, -1.6418) centre (-2.4252, 2.0921) ccw
  arc A369 (-6.1468, -1.6418) -> (-5.8594, -1.9113) centre (-1.6229, 2.8962) ccw
  arc A370 (-5.8594, -1.9113) -> (-5.4845, -2.2208) centre (-0.8427, 3.7809) ccw
  arc A371 (-5.4845, -2.2208) -> (-5.136, -2.0257) centre (-15.3265, 15.7621) ccw
  arc A372 (-5.136, -2.0257) -> (-5.2041, -1.5443) centre (-12.6787, -2.8476) ccw
  arc A373 (-5.2041, -1.5443) -> (-5.2837, -1.1585) centre (-11.5167, -2.6446) ccw
  arc A374 (-5.2837, -1.1585) -> (-5.3653, -0.8561) centre (-10.412, -2.3807) ccw
  arc A375 (-5.3653, -0.8561) -> (-5.0419, -0.658) centre (-15.3265, 15.7621) ccw
  arc A376 (-5.0419, -0.658) -> (-4.8096, -0.868) centre (-1.3924, 3.1465) ccw
  arc A377 (-4.8096, -0.868) -> (-4.5019, -1.114) centre (-0.6557, 4.011) ccw
  arc A378 (-4.5019, -1.114) -> (-4.104, -1.3932) centre (0.0527, 4.9542) ccw
  arc A379 (-4.104, -1.3932) -> (-3.7718, -1.1713) centre (-15.3265, 15.7621) ccw
  arc A380 (-3.7718, -1.1713) -> (-3.8775, -0.6968) centre (-11.2268, -2.5825) ccw
  arc A381 (-3.8775, -0.6968) -> (-3.9871, -0.3184) centre (-10.0843, -2.2889) ccw
  arc A382 (-3.9871, -0.3184) -> (-4.0922, -0.0233) centre (-9.0037, -1.9392) ccw
  arc A383 (-4.0922, -0.0233) -> (-3.7853, 0.1996) centre (-15.3265, 15.7621) ccw
  arc A384 (-3.7853, 0.1996) -> (-3.5372, 0.0085) centre (-0.4455, 4.2787) ccw
  arc A385 (-3.5372, 0.0085) -> (-3.2112, -0.2127) centre (0.221, 5.1983) ccw
  arc A386 (-3.2112, -0.2127) -> (-2.7926, -0.4598) centre (0.8532, 6.1942) ccw
  arc A387 (-2.7926, -0.4598) -> (-2.4789, -0.2125) centre (-15.3265, 15.7621) ccw
  arc A388 (-2.4789, -0.2125) -> (-2.6214, 0.2522) centre (-9.8001, -2.2042) ccw
  arc A389 (-2.6214, 0.2522) -> (-2.7604, 0.6209) centre (-8.6842, -1.822) ccw
  arc A390 (-2.7604, 0.6209) -> (-2.8883, 0.9068) centre (-7.6343, -1.3885) ccw
  arc A391 (-2.8883, 0.9068) -> (-2.5999, 1.1531) centre (-15.3265, 15.7621) ccw
  arc A392 (-2.5999, 1.1531) -> (-2.3376, 0.982) centre (0.4096, 5.4816) ccw
  arc A393 (-2.3376, 0.982) -> (-1.9952, 0.7871) centre (1.0019, 6.4507) ccw
  arc A394 (-1.9952, 0.7871) -> (-1.5585, 0.5736) centre (1.554, 7.4931) ccw
  arc A395 (-1.5585, 0.5736) -> (-1.2651, 0.8447) centre (-15.3265, 15.7621) ccw
  arc A396 (-1.2651, 0.8447) -> (-1.4437, 1.2969) centre (-8.4075, -1.7153) ccw
  arc A397 (-1.4437, 1.2969) -> (-1.6111, 1.6535) centre (-7.325, -1.2466) ccw
  arc A398 (-1.6111, 1.6535) -> (-1.7611, 1.9284) centre (-6.3124, -0.7321) ccw
  arc A399 (-1.7611, 1.9284) -> (-1.4929, 2.1966) centre (-15.3265, 15.7621) ccw
  arc A400 (-1.4929, 2.1966) -> (-1.218, 2.0467) centre (1.1676, 6.7479) ccw
  arc A401 (-1.218, 2.0467) -> (-0.8613, 1.8792) centre (1.6821, 7.7605) ccw
  arc A402 (-0.8613, 1.8792) -> (-0.4092, 1.7006) centre (2.1508, 8.843) ccw
  arc A403 (-0.4092, 1.7006) -> (-0.1381, 1.994) centre (-15.3265, 15.7621) ccw
  arc A404 (-0.1381, 1.994) -> (-0.3516, 2.4307) centre (-7.0576, -1.1185) ccw
  arc A405 (-0.3516, 2.4307) -> (-0.5465, 2.7731) centre (-6.0152, -0.5664) ccw
  arc A406 (-0.5465, 2.7731) -> (-0.7175, 3.0354) centre (-5.0461, 0.026) ccw
  arc A407 (-0.7175, 3.0354) -> (-0.4712, 3.3238) centre (-15.3265, 15.7621) ccw
  arc A408 (-0.4712, 3.3238) -> (-0.1854, 3.1959) centre (1.824, 8.0698) ccw
  arc A409 (-0.1854, 3.1959) -> (0.1833, 3.057) centre (2.2575, 9.1197) ccw
  arc A410 (0.1833, 3.057) -> (0.648, 2.9144) centre (2.6398, 10.2356) ccw
  arc A411 (0.648, 2.9144) -> (0.8953, 3.2281) centre (-15.3265, 15.7621) ccw
  arc A412 (0.8953, 3.2281) -> (0.6482, 3.6467) centre (-5.7587, -0.4177) ccw
  arc A413 (0.6482, 3.6467) -> (0.4271, 3.9728) centre (-4.7628, 0.2145) ccw
  arc A414 (0.4271, 3.9728) -> (0.236, 4.2209) centre (-3.8431, 0.8811) ccw
  arc A415 (0.236, 4.2209) -> (0.4589, 4.5277) centre (-15.3265, 15.7621) ccw
  arc A416 (0.4589, 4.5277) -> (0.7539, 4.4226) centre (2.3747, 9.4392) ccw
  arc A417 (0.7539, 4.4226) -> (1.1323, 4.313) centre (2.7245, 10.5198) ccw
  arc A418 (1.1323, 4.313) -> (1.6068, 4.2073) centre (3.018, 11.6623) ccw
  arc A419 (1.6068, 4.2073) -> (1.8287, 4.5395) centre (-15.3265, 15.7621) ccw
  arc A420 (1.8287, 4.5395) -> (1.5495, 4.9374) centre (-4.5187, 0.3829) ccw
  arc A421 (1.5495, 4.9374) -> (1.3035, 5.2451) centre (-3.5755, 1.0913) ccw
  arc A422 (1.3035, 5.2451) -> (1.0935, 5.4775) centre (-2.711, 1.8279) ccw
  arc A423 (1.0935, 5.4775) -> (1.2916, 5.8008) centre (-15.3265, 15.7621) ccw
  arc A424 (1.2916, 5.8008) -> (1.594, 5.7192) centre (2.8162, 10.8475) ccw
  arc A425 (1.594, 5.7192) -> (1.9799, 5.6397) centre (3.0801, 11.9522) ccw
  arc A426 (1.9799, 5.6397) -> (2.4612, 5.5715) centre (3.2831, 13.1142) ccw
  arc A427 (2.4612, 5.5715) -> (2.6564, 5.9201) centre (-15.3265, 15.7621) ccw
  arc A428 (2.6564, 5.9201) -> (2.3468, 6.2949) centre (-3.3454, 1.2782) ccw
  arc A429 (2.3468, 6.2949) -> (2.0774, 6.5823) centre (-2.4606, 2.0585) ccw
  arc A430 (2.0774, 6.5823) -> (1.8498, 6.7975) centre (-1.6566, 2.8607) ccw
  arc A431 (1.8498, 6.7975) -> (2.022, 7.1354) centre (-15.3265, 15.7621) ccw
  arc A432 (2.022, 7.1354) -> (2.3298, 7.0777) centre (3.1459, 12.2861) ccw
  arc A433 (2.3298, 7.0777) -> (2.7207, 7.0287) centre (3.3223, 13.4081) ccw
  arc A434 (2.7207, 7.0287) -> (3.2059, 6.9986) centre (3.4335, 14.5825) ccw
  arc A435 (3.2059, 6.9986) -> (3.3731, 7.3613) centre (-15.3265, 15.7621) ccw
  arc A436 (3.3731, 7.3613) -> (3.0351, 7.7107) centre (-2.2459, 2.2629) ccw
  arc A437 (3.0351, 7.7107) -> (2.7439, 7.9761) centre (-1.4251, 3.1101) ccw
  arc A438 (2.7439, 7.9761) -> (2.5002, 8.1727) centre (-0.6865, 3.973) ccw
  arc A439 (2.5002, 8.1727) -> (2.6453, 8.5231) centre (-15.3265, 15.7621) ccw
  arc A440 (2.6453, 8.5231) -> (2.9567, 8.4898) centre (3.3617, 13.7462) ccw
  arc A441 (2.9567, 8.4898) -> (3.3503, 8.4716) centre (3.4495, 14.8785) ccw
  arc A442 (3.3503, 8.4716) -> (3.8363, 8.4796) centre (3.4682, 16.058) ccw
  arc A443 (3.8363, 8.4796) -> (3.9746, 8.8544) centre (-15.3265, 15.7621) ccw
  arc A444 (3.9746, 8.8544) -> (3.6102, 9.1762) centre (-1.2271, 3.3308) ccw
  arc A445 (3.6102, 9.1762) -> (3.2991, 9.4179) centre (-0.4753, 4.2398) ccw
  arc A446 (3.2991, 9.4179) -> (3.0407, 9.5948) centre (0.1933, 5.158) ccw
  arc A447 (3.0407, 9.5948) -> (3.1579, 9.9555) centre (-15.3265, 15.7621) ccw
  arc A448 (3.1579, 9.9555) -> (3.4709, 9.9467) centre (3.4622, 15.2186) ccw
  arc A449 (3.4709, 9.9467) -> (3.8647, 9.9594) centre (3.4609, 16.3544) ccw
  arc A450 (3.8647, 9.9594) -> (4.3486, 10.0056) centre (3.387, 17.5317) ccw
  arc A451 (4.3486, 10.0056) -> (4.4571, 10.39) centre (-15.3265, 15.7621) ccw
  arc A452 (4.4571, 10.39) -> (4.0686, 10.6822) centre (-0.2952, 4.4754) ccw
  arc A453 (4.0686, 10.6822) -> (3.7395, 10.8988) centre (0.3829, 5.4406) ccw
  arc A454 (3.7395, 10.8988) -> (3.468, 11.0549) centre (0.9775, 6.4083) ccw
  arc A455 (3.468, 11.0549) -> (3.5565, 11.4237) centre (-15.3265, 15.7621) ccw
  arc A456 (3.5565, 11.4237) -> (3.8693, 11.4395) centre (3.4469, 16.6945) ccw
  arc A457 (3.8693, 11.4395) -> (4.2608, 11.4831) centre (3.3565, 17.8266) ccw
  arc A458 (4.2608, 11.4831) -> (4.7396, 11.567) centre (3.1905, 18.9945) ccw
  arc A459 (4.7396, 11.567) -> (4.8176, 11.9588) centre (-15.3265, 15.7621) ccw
  arc A460 (4.8176, 11.9588) -> (4.4073, 12.2196) centre (0.544, 5.6895) ccw
  arc A461 (4.4073, 12.2196) -> (4.0622, 12.4097) centre (1.1443, 6.7049) ccw
  arc A462 (4.0622, 12.4097) -> (3.7793, 12.544) centre (1.6611, 7.7164) ccw
  arc A463 (3.7793, 12.544) -> (3.8387, 12.9186) centre (-15.3265, 15.7621) ccw
  arc A464 (3.8387, 12.9186) -> (4.1492, 12.9589) centre (3.3159, 18.1645) ccw
  arc A465 (4.1492, 12.9589) -> (4.5362, 13.033) centre (3.137, 19.2861) ccw
  arc A466 (4.5362, 13.033) -> (5.0069, 13.1543) centre (2.8798, 20.4374) ccw
  arc A467 (5.0069, 13.1543) -> (5.0539, 13.551) centre (-15.3265, 15.7621) ccw
  arc A468 (5.0539, 13.551) -> (4.6244, 13.7788) centre (1.2853, 6.9657) ccw
  arc A469 (4.6244, 13.7788) -> (4.2655, 13.9413) centre (1.8041, 8.0251) ccw
  arc A470 (4.2655, 13.9413) -> (3.9729, 14.053) centre (2.24, 9.074) ccw
  arc A471 (3.9729, 14.053) -> (4.0027, 14.431) centre (-15.3265, 15.7621) ccw
  arc A472 (4.0027, 14.431) -> (4.3091, 14.4956) centre (3.0699, 19.6198) ccw
  arc A473 (4.3091, 14.4956) -> (4.6891, 14.5999) centre (2.8036, 20.7239) ccw
  arc A474 (4.6891, 14.5999) -> (5.1488, 14.7577) centre (2.4569, 21.8514) ccw
  arc A475 (5.1488, 14.7577) -> (5.1645, 15.1569) centre (-15.3265, 15.7621) ccw
  arc A476 (5.1645, 15.1569) -> (4.7185, 15.3503) centre (1.9243, 8.2962) ccw
  arc A477 (4.7185, 15.3503) -> (4.348, 15.4841) centre (2.3584, 9.3931) ccw
  arc A478 (4.348, 15.4841) -> (4.0475, 15.5724) centre (2.7106, 10.4729) ccw
  arc A479 (4.0475, 15.5724) -> (4.0475, 15.9517) centre (-15.3265, 15.7621) ccw
  arc A480 (4.0475, 15.9517) -> (4.348, 16.0401) centre (2.7106, 21.0513) ccw
  arc A481 (4.348, 16.0401) -> (4.7185, 16.1739) centre (2.3584, 22.1311) ccw
  arc A482 (4.7185, 16.1739) -> (5.1645, 16.3673) centre (1.9243, 23.2279) ccw
  arc A483 (5.1645, 16.3673) -> (5.1488, 16.7664) centre (-15.3265, 15.7621) ccw
  arc A484 (5.1488, 16.7664) -> (4.6891, 16.9243) centre (2.4569, 9.6727) ccw
  arc A485 (4.6891, 16.9243) -> (4.3091, 17.0286) centre (2.8036, 10.8002) ccw
  arc A486 (4.3091, 17.0286) -> (4.0027, 17.0931) centre (3.0699, 11.9043) ccw
  arc A487 (4.0027, 17.0931) -> (3.9729, 17.4712) centre (-15.3265, 15.7621) ccw
  arc A488 (3.9729, 17.4712) -> (4.2655, 17.5829) centre (2.24, 22.4501) ccw
  arc A489 (4.2655, 17.5829) -> (4.6244, 17.7453) centre (1.8041, 23.499) ccw
  arc A490 (4.6244, 17.7453) -> (5.0539, 17.9731) centre (1.2853, 24.5584) ccw
  arc A491 (5.0539, 17.9731) -> (5.0069, 18.3698) centre (-15.3265, 15.7621) ccw
  arc A492 (5.0069, 18.3698) -> (4.5362, 18.4911) centre (2.8798, 11.0868) ccw
  arc A493 (4.5362, 18.4911) -> (4.1492, 18.5653) centre (3.137, 12.238) ccw
  arc A494 (4.1492, 18.5653) -> (3.8387, 18.6055) centre (3.3159, 13.3596) ccw
  arc A495 (3.8387, 18.6055) -> (3.7793, 18.9801) centre (-15.3265, 15.7621) ccw
  arc A496 (3.7793, 18.9801) -> (4.0622, 19.1144) centre (1.6611, 23.8078) ccw
  arc A497 (4.0622, 19.1144) -> (4.4073, 19.3045) centre (1.1443, 24.8192) ccw
  arc A498 (4.4073, 19.3045) -> (4.8176, 19.5653) centre (0.544, 25.8346) ccw
  arc A499 (4.8176, 19.5653) -> (4.7396, 19.9571) centre (-15.3265, 15.7621) ccw
  arc A500 (4.7396, 19.9571) -> (4.2608, 20.0411) centre (3.1905, 12.5296) ccw
  arc A501 (4.2608, 20.0411) -> (3.8693, 20.0847) centre (3.3565, 13.6975) ccw
  arc A502 (3.8693, 20.0847) -> (3.5565, 20.1005) centre (3.4469, 14.8297) ccw
  arc A503 (3.5565, 20.1005) -> (3.468, 20.4692) centre (-15.3265, 15.7621) ccw
  arc A504 (3.468, 20.4692) -> (3.7395, 20.6253) centre (0.9775, 25.1158) ccw
  arc A505 (3.7395, 20.6253) -> (4.0686, 20.8419) centre (0.3829, 26.0836) ccw
  arc A506 (4.0686, 20.8419) -> (4.4571, 21.1341) centre (-0.2952, 27.0488) ccw
  arc A507 (4.4571, 21.1341) -> (4.3486, 21.5186) centre (-15.3265, 15.7621) ccw
  arc A508 (4.3486, 21.5186) -> (3.8647, 21.5647) centre (3.387, 13.9924) ccw
  arc A509 (3.8647, 21.5647) -> (3.4709, 21.5774) centre (3.4609, 15.1697) ccw
  arc A510 (3.4709, 21.5774) -> (3.1579, 21.5686) centre (3.4622, 16.3055) ccw
  arc A511 (3.1579, 21.5686) -> (3.0407, 21.9293) centre (-15.3265, 15.7621) ccw
  arc A512 (3.0407, 21.9293) -> (3.2991, 22.1062) centre (0.1933, 26.3662) ccw
  arc A513 (3.2991, 22.1062) -> (3.6102, 22.348) centre (-0.4753, 27.2843) ccw
  arc A514 (3.6102, 22.348) -> (3.9746, 22.6697) centre (-1.2271, 28.1933) ccw
  arc A515 (3.9746, 22.6697) -> (3.8363, 23.0445) centre (-15.3265, 15.7621) ccw
  arc A516 (3.8363, 23.0445) -> (3.3503, 23.0525) centre (3.4682, 15.4661) ccw
  arc A517 (3.3503, 23.0525) -> (2.9567, 23.0343) centre (3.4495, 16.6456) ccw
  arc A518 (2.9567, 23.0343) -> (2.6453, 23.001) centre (3.3617, 17.778) ccw
  arc A519 (2.6453, 23.001) -> (2.5002, 23.3514) centre (-15.3265, 15.7621) ccw
  arc A520 (2.5002, 23.3514) -> (2.7439, 23.548) centre (-0.6865, 27.5512) ccw
  arc A521 (2.7439, 23.548) -> (3.0351, 23.8134) centre (-1.4251, 28.414) ccw
  arc A522 (3.0351, 23.8134) -> (3.3731, 24.1628) centre (-2.2459, 29.2612) ccw
  arc A523 (3.3731, 24.1628) -> (3.2059, 24.5256) centre (-15.3265, 15.7621) ccw
  arc A524 (3.2059, 24.5256) -> (2.7207, 24.4954) centre (3.4335, 16.9417) ccw
  arc A525 (2.7207, 24.4954) -> (2.3298, 24.4464) centre (3.3223, 18.116) ccw
  arc A526 (2.3298, 24.4464) -> (2.022, 24.3888) centre (3.1459, 19.238) ccw
  arc A527 (2.022, 24.3888) -> (1.8498, 24.7267) centre (-15.3265, 15.7621) ccw
  arc A528 (1.8498, 24.7267) -> (2.0774, 24.9418) centre (-1.6566, 28.6635) ccw
  arc A529 (2.0774, 24.9418) -> (2.3468, 25.2293) centre (-2.4606, 29.4657) ccw
  arc A530 (2.3468, 25.2293) -> (2.6564, 25.6041) centre (-3.3454, 30.2459) ccw
  arc A531 (2.6564, 25.6041) -> (2.4612, 25.9526) centre (-15.3265, 15.7621) ccw
  arc A532 (2.4612, 25.9526) -> (1.9799, 25.8845) centre (3.2831, 18.4099) ccw
  arc A533 (1.9799, 25.8845) -> (1.594, 25.8049) centre (3.0801, 19.5719) ccw
  arc A534 (1.594, 25.8049) -> (1.2916, 25.7233) centre (2.8162, 20.6766) ccw
  arc A535 (1.2916, 25.7233) -> (1.0935, 26.0467) centre (-15.3265, 15.7621) ccw
  arc A536 (1.0935, 26.0467) -> (1.3035, 26.279) centre (-2.711, 29.6962) ccw
  arc A537 (1.3035, 26.279) -> (1.5495, 26.5867) centre (-3.5755, 30.4329) ccw
  arc A538 (1.5495, 26.5867) -> (1.8287, 26.9846) centre (-4.5187, 31.1413) ccw
  arc A539 (1.8287, 26.9846) -> (1.6068, 27.3168) centre (-15.3265, 15.7621) ccw
  arc A540 (1.6068, 27.3168) -> (1.1323, 27.2111) centre (3.018, 19.8618) ccw
  arc A541 (1.1323, 27.2111) -> (0.7539, 27.1015) centre (2.7245, 21.0044) ccw
  arc A542 (0.7539, 27.1015) -> (0.4589, 26.9964) centre (2.3747, 22.085) ccw
  arc A543 (0.4589, 26.9964) -> (0.236, 27.3033) centre (-15.3265, 15.7621) ccw
  arc A544 (0.236, 27.3033) -> (0.4271, 27.5514) centre (-3.8431, 30.6431) ccw
  arc A545 (0.4271, 27.5514) -> (0.6482, 27.8774) centre (-4.7628, 31.3096) ccw
  arc A546 (0.6482, 27.8774) -> (0.8953, 28.296) centre (-5.7587, 31.9418) ccw
  arc A547 (0.8953, 28.296) -> (0.648, 28.6097) centre (-15.3265, 15.7621) ccw
  arc A548 (0.648, 28.6097) -> (0.1833, 28.4672) centre (2.6398, 21.2885) ccw
  arc A549 (0.1833, 28.4672) -> (-0.1854, 28.3282) centre (2.2575, 22.4045) ccw
  arc A550 (-0.1854, 28.3282) -> (-0.4712, 28.2003) centre (1.824, 23.4543) ccw
  arc A551 (-0.4712, 28.2003) -> (-0.7175, 28.4887) centre (-15.3265, 15.7621) ccw
  arc A552 (-0.7175, 28.4887) -> (-0.5465, 28.751) centre (-5.0461, 31.4982) ccw
  arc A553 (-0.5465, 28.751) -> (-0.3516, 29.0934) centre (-6.0152, 32.0905) ccw
  arc A554 (-0.3516, 29.0934) -> (-0.1381, 29.5302) centre (-7.0576, 32.6427) ccw
  arc A555 (-0.1381, 29.5302) -> (-0.4092, 29.8235) centre (-15.3265, 15.7621) ccw
  arc A556 (-0.4092, 29.8235) -> (-0.8613, 29.6449) centre (2.1508, 22.6811) ccw
  arc A557 (-0.8613, 29.6449) -> (-1.218, 29.4775) centre (1.6821, 23.7636) ccw
  arc A558 (-1.218, 29.4775) -> (-1.4929, 29.3275) centre (1.1676, 24.7762) ccw
  arc A559 (-1.4929, 29.3275) -> (-1.7611, 29.5957) centre (-15.3265, 15.7621) ccw
  arc A560 (-1.7611, 29.5957) -> (-1.6111, 29.8706) centre (-6.3124, 32.2563) ccw